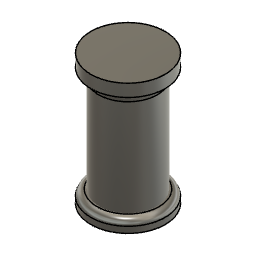
Pins (Autodesk Fusion 360 design; units mm, degrees)
Autodesk Fusion 360 part; units mm, degrees
note: some values were not read from the file. Chosen so that the rebuilt part matches the saved one: which bodies a step acts on.
sketch "Initial" plane through (0, 0, 0) normal (0, 1, 0) x (1, 0, 0) in component "Pin Body"
  circle A0 centre (0, 0) radius 4.75
  circle A1 centre (0, 0) radius 2.375
  dimension "d1" = 9.5
  dimension "d4" = 4.75
  constraint coincident A0.centre A1.centre
  constraint concentric A0 A1
  measures "d1" diameter of A0
  measures "d4" diameter of A1
extrude "Extrude1" add sketch "Initial" along normal blind 19 contours A0 | A1 makes body 1 in component "Pin Body"
extrude "Extrude2" add sketch "Initial" along normal blind 10 contours A1 bodies 1 in component "Pin Body"
split "Split1" by curves path "Initial" along A1 bodies 1 makes body 2 at (4.7264, 12.6667, 0.4729) in component "Pin Body"
sketch "Inner" plane through (0, 0, 0) normal (0, 1, 0) x (1, 0, 0) in component "Pin Body"
  circle A0 centre (0, 0) radius 6
  dimension "d9" = 12
  constraint coincident A0.centre origin
  measures "d9" diameter of A0
extrude "Extrude3" add sketch "Inner" along normal blind 2 bodies 1 in component "Pin Body"
fillet "Fillet2" radius 1 1 edges at (-5.594, 2, 2.1697) on bodies 1 in component "Pin Body"
sketch "Sketch3" plane through (0, 19, 0) normal (0, 1, 0) x (-1, 0, 0) in component "Pin Body"
  circle A0 centre (0, 0) radius 2.375
  circle A1 centre (0, 0) radius 4.75
  circle A2 centre (0, 0) radius 6
  dimension "d14" = 12
  constraint concentric A0 A2
  measures "d14" diameter of A2
extrude "Extrude4" add sketch "Sketch3" along normal blind 2 contours A0 | A1 | A2 bodies 2 in component "Pin Body"
fillet "Fillet4" radius 1.5 1 edges at (-4.4286, 19, 1.7177) on bodies 2 in component "Pin Body"
sketch "Sketch4" plane through (0, 19, 0) normal (0, 1, 0) x (-1, 0, 0) in component "Pin Body"
  circle A0 centre (0, 0) radius 2.375
  circle A1 centre (0, 0) radius 2.225
  dimension "d21" = -0.15
extrude "Extrude5" cut sketch "Sketch4" against normal up to surface (17 mm away) bodies 1 in component "Pin Body"
fillet "Fillet5" radius 1.5 1 faces at (0.4378, 19, -0.5371) on bodies 1 in component "Pin Body"
component "Pin Body" placed x (1, 0, 0) y (0, 1, 0) z (0, 0, 1) at (0, 0, 0)
named bodies: "Bot", "Top"
